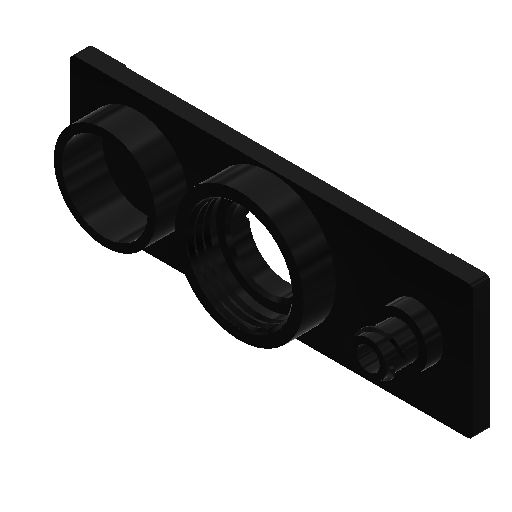
# Autodesk Inventor part: PRT - 9301 - MFLEAFCHIP - V04 - A
Saved by Autodesk Inventor 2025.3 (Build 293356000, 356)
## iProperties
Part Number: PRT - 9301 - MFLEAFCHIP - V04 - A
Material: Generic
Description: Leaf chamber chip A (luer inlet -> chamber -> open reservoir), print in black resin
Document SubType Name: Modeling
Designer: benir
Appearance: Low Gloss - Black
Author: benir
Autodesk Inventor part; units mm, degrees
ref_plane "z = -cs_recess" through (0, 0, -0.25) normal (0, 0, 1) x (1, 0, 0)
sketch "slab sketch" plane through (0, 0, -0.25) normal (0, 0, 1) x (1, 0, 0)
  line L0 (-37.5, -12.5) -> (37.5, -12.5)
  line L1 (37.5, -12.5) -> (37.5, 12.5)
  line L2 (37.5, 12.5) -> (-37.5, 12.5)
  line L3 (-37.5, 12.5) -> (-37.5, -12.5)
  line L4 (0, -17.5) -> (0, 17.5) projected
  line L5 (-52.5, 0) -> (52.5, 0) projected
  dimension "d1" = 75
  dimension "d2" = 25
  constraints: 8 end point, 2 parallel, 1 horizontal, 1 perpendicular, 2 other
  measures "d1" distance of L0.start L0.end
  measures "d2" distance of L2.end L0.start
extrude "slab" add sketch "slab sketch" along normal blind 3.25
fillet "slab corners" radius 1 4 edges at (-37.5, -12.5, 1.375) (-37.5, 12.5, 1.375) (37.5, 12.5, 1.375) (37.5, -12.5, 1.375)
sketch "glue band sketch" plane through (0, 0, 0) normal (0, 0, 1) x (1, 0, 0)
  line L0 (-30.25, -13.5) -> (30.25, -13.5)
  line L1 (30.25, -13.5) -> (30.25, 13.5)
  line L2 (30.25, 13.5) -> (-30.25, 13.5)
  line L3 (-30.25, 13.5) -> (-30.25, -13.5)
  line L4 (0, -18.9) -> (0, 18.9) projected
  line L5 (-52.5, 0) -> (52.5, 0) projected
  dimension "d6" = 60.5
  dimension "d7" = 27
  constraints: 8 end point, 2 parallel, 1 horizontal, 1 perpendicular, 2 other
  measures "d6" distance of L0.start L0.end
  measures "d7" distance of L2.end L0.start
extrude "glue band (bottom coverslip)" cut sketch "glue band sketch" against normal blind 0.75
ref_plane "z = base_t" through (0, 0, 3) normal (0, 0, 1) x (1, 0, 0)
sketch "chamber boss sketch" plane through (0, 0, 3) normal (0, 0, 1) x (1, 0, 0)
  circle A0 centre (0, 0) radius 12
  dimension "d11" = 24
  constraints: 1 centre point
  measures "d11" diameter of A0
extrude "chamber boss" add sketch "chamber boss sketch" along normal blind 6
sketch "reservoir boss sketch" plane through (0, 0, 3) normal (0, 0, 1) x (1, 0, 0)
  circle A0 centre (-25, 0) radius 9.5
  line L0 (-52.5, 0) -> (52.5, 0) projected
  point P0 (0, 0)
  dimension "d14" = 25
  dimension "d15" = 19
  constraints: 1 centre point, 1 point on line
  measures "d14" distance of point (0, 0) A0.centre
  measures "d15" diameter of A0
extrude "reservoir boss" add sketch "reservoir boss sketch" along normal blind 6
sketch "inlet luer foot sketch" plane through (0, 0, 3) normal (0, 0, 1) x (1, 0, 0)
  circle A0 centre (27, 0) radius 5
  line L0 (-52.5, 0) -> (52.5, 0) projected
  point P0 (0, 0)
  dimension "d18" = 27
  dimension "d19" = 10
  constraints: 1 centre point, 1 point on line
  measures "d18" distance of point (0, 0) A0.centre
  measures "d19" diameter of A0
extrude "inlet luer foot" add sketch "inlet luer foot sketch" along normal blind 3
sketch "inlet luer hub sketch" plane through (0, 0, 3) normal (0, 0, 1) x (1, 0, 0)
  circle A0 centre (27, 0) radius 3.365
  line L0 (-52.5, 0) -> (52.5, 0) projected
  point P0 (0, 0)
  dimension "d22" = 27
  dimension "d23" = 6.73
  constraints: 1 centre point, 1 point on line
  measures "d22" distance of point (0, 0) A0.centre
  measures "d23" diameter of A0
extrude "inlet luer hub" add sketch "inlet luer hub sketch" along normal blind 9
ref_plane "x = in_x" through (27, 0, 0) normal (1, 0, 0) x (0, 1, 0)
sketch "inlet luer lug profile" plane through (0, 0, 0) normal (0, 1, 0) x (-1, 0, 0)
  line L0 (-30.265, 8.25) -> (-30.915, 8.55)
  line L1 (-30.915, 8.55) -> (-30.915, 8.9)
  line L2 (-30.915, 8.9) -> (-30.265, 9.2)
  line L3 (-30.265, 9.2) -> (-30.265, 8.25)
  point P0 (0, 0)
  dimension "d27" = 8.25
  dimension "d28" = 30.265
  dimension "d29" = 8.55
  dimension "d30" = 30.915
  dimension "d31" = 8.9
  dimension "d32" = 30.915
  dimension "d33" = 9.2
  dimension "d34" = 30.265
  constraints: 8 end point
  measures "d27" vertical distance of point (0, 0) L0.start
  measures "d28" horizontal distance of point (0, 0) L0.start
  measures "d29" vertical distance of point (0, 0) L0.end
  measures "d30" horizontal distance of point (0, 0) L0.end
  measures "d31" vertical distance of point (0, 0) L1.end
  measures "d32" horizontal distance of point (0, 0) L1.end
  measures "d33" vertical distance of point (0, 0) L2.end
  measures "d34" horizontal distance of point (0, 0) L2.end
coil "inlet luer lug (RH, lead luer_lead)" sketch "inlet luer lug profile" operation add axis through (27, 0, 0) along (0, 0, 1) pitch 5 turns 0.5 hand right
pattern_circular "inlet luer lugs x2" count 2 over 360 about axis through (27, 0, 0) along (0, 0, 1) of "inlet luer lug (RH, lead luer_lead)"
sketch "well sketch" plane through (0, 0, 0) normal (0, 0, 1) x (1, 0, 0)
  circle A0 centre (0, 0) radius 7.15
  dimension "d46" = 14.3
  constraints: 1 centre point
  measures "d46" diameter of A0
extrude "chamber well" cut sketch "well sketch" along normal blind 4
ref_plane "z = ledge_z" through (0, 0, 4) normal (0, 0, 1) x (1, 0, 0)
sketch "thread bore sketch" plane through (0, 0, 4) normal (0, 0, 1) x (1, 0, 0)
  circle A0 centre (0, 0) radius 9.338125
  dimension "d50" = 18.67625
  constraints: 1 centre point
  measures "d50" diameter of A0
extrude "thread bore" cut sketch "thread bore sketch" along normal blind 6
chamfer "thread lead-in" distance 0.6 angle 45 1 edges at (-9.3381, 0, 9)
chamfer "O-ring lead-in" distance 0.6 angle 45 1 edges at (-7.15, 0, 4)
sketch "internal thread groove profile" plane through (0, 0, 0) normal (0, 1, 0) x (-1, 0, 0)
  line L0 (-9.238125, 4.3) -> (-10.15, 4.826471)
  line L1 (-10.15, 4.826471) -> (-10.15, 5.013971)
  line L2 (-10.15, 5.013971) -> (-9.238125, 5.540442)
  line L3 (-9.238125, 5.540442) -> (-9.238125, 4.3)
  point P0 (0, 0)
  dimension "d59" = 4.3
  dimension "d60" = 9.23813
  dimension "d61" = 4.82647
  dimension "d62" = 10.15
  dimension "d63" = 5.01397
  dimension "d64" = 10.15
  dimension "d65" = 5.54044
  dimension "d66" = 9.23813
  constraints: 8 end point
  measures "d59" vertical distance of point (0, 0) L0.start
  measures "d60" horizontal distance of point (0, 0) L0.start
  measures "d61" vertical distance of point (0, 0) L0.end
  measures "d62" horizontal distance of point (0, 0) L0.end
  measures "d63" vertical distance of point (0, 0) L1.end
  measures "d64" horizontal distance of point (0, 0) L1.end
  measures "d65" vertical distance of point (0, 0) L2.end
  measures "d66" horizontal distance of point (0, 0) L2.end
coil "M20x1.5 internal thread (coil cut, RH)" sketch "internal thread groove profile" operation cut axis through (0, 0, -10) along (0, 0, 1) pitch 1.5 turns 3.719853 hand right
ref_plane "z = res_top" through (0, 0, 9) normal (0, 0, 1) x (1, 0, 0)
sketch "reservoir sketch" plane through (0, 0, 9) normal (0, 0, 1) x (1, 0, 0)
  circle A0 centre (-25, 0) radius 8
  line L0 (-52.5, 0) -> (52.5, 0) projected
  point P0 (0, 0)
  dimension "d76" = 25
  dimension "d77" = 16
  constraints: 1 centre point, 1 point on line
  measures "d76" distance of point (0, 0) A0.centre
  measures "d77" diameter of A0
extrude "reservoir" cut sketch "reservoir sketch" against normal blind 7.5
ref_plane "z = luer_top" through (0, 0, 12) normal (0, 0, 1) x (1, 0, 0)
sketch "inlet luer bore sketch" plane through (0, 0, 12) normal (0, 0, 1) x (1, 0, 0)
  circle A0 centre (27, 0) radius 2.145
  line L0 (-52.5, 0) -> (52.5, 0) projected
  point P0 (0, 0)
  dimension "d81" = 27
  dimension "d82" = 4.29
  constraints: 1 centre point, 1 point on line
  measures "d81" distance of point (0, 0) A0.centre
  measures "d82" diameter of A0
sketch "inlet luer bore sketch outline for inlet luer taper bore (6 %)" plane through (0, 0, 12) normal (0, 0, 1) x (1, 0, 0)
  circle A0 centre (27, 0) radius 2.145
extrude "inlet luer taper bore (6 %)" cut sketch "inlet luer bore sketch outline for inlet luer taper bore (6 %)" against normal blind 8 draft -1.71836
ref_plane "z = ch_floor" through (0, 0, 0) normal (0, 0, 1) x (1, 0, 0)
sketch "channel sketch" plane through (0, 0, 0) normal (0, 0, 1) x (1, 0, 0)
  line L0 (3.575, -0.5) -> (27, -0.5)
  line L1 (27, -0.5) -> (27, 0.5)
  line L2 (27, 0.5) -> (3.575, 0.5)
  line L3 (3.575, 0.5) -> (3.575, -0.5)
  line L4 (-52.5, 0) -> (52.5, 0) projected
  line L5 (-25, -0.5) -> (-3.575, -0.5)
  line L6 (-3.575, -0.5) -> (-3.575, 0.5)
  line L7 (-3.575, 0.5) -> (-25, 0.5)
  line L8 (-25, 0.5) -> (-25, -0.5)
  point P0 (0, 0)
  dimension "d86" = 1
  dimension "d87" = 3.575
  dimension "d88" = 27
  dimension "d89" = 1
  dimension "d90" = 25
  dimension "d91" = 3.575
  constraints: 16 end point, 4 parallel, 2 horizontal, 2 perpendicular, 2 other
  measures "d86" distance of L2.end L0.start
  measures "d87" horizontal distance of point (0, 0) L2.end
  measures "d88" horizontal distance of point (0, 0) L0.end
  measures "d89" distance of L7.end L5.start
  measures "d90" horizontal distance of point (0, 0) L7.end
  measures "d91" horizontal distance of point (0, 0) L5.end
extrude "channels" cut sketch "channel sketch" along normal blind 0.5
sketch "inlet via sketch" plane through (0, 0, 0) normal (0, 0, 1) x (1, 0, 0)
  circle A0 centre (27, 0) radius 0.5
  line L0 (-52.5, 0) -> (52.5, 0) projected
  point P0 (0, 0)
  dimension "d94" = 27
  dimension "d95" = 1
  constraints: 1 centre point, 1 point on line
  measures "d94" distance of point (0, 0) A0.centre
  measures "d95" diameter of A0
extrude "inlet via" cut sketch "inlet via sketch" along normal blind 4.3
sketch "outlet via sketch" plane through (0, 0, 0) normal (0, 0, 1) x (1, 0, 0)
  circle A0 centre (-25, 0) radius 0.5
  line L0 (-52.5, 0) -> (52.5, 0) projected
  point P0 (0, 0)
  dimension "d98" = 25
  dimension "d99" = 1
  constraints: 1 centre point, 1 point on line
  measures "d98" distance of point (0, 0) A0.centre
  measures "d99" diameter of A0
extrude "outlet via" cut sketch "outlet via sketch" along normal blind 1.8
equation "\"d1\" = chip_l"
equation "\"d2\" = chip_w"
equation "\"d3\" = base_t + cs_recess"
equation "\"d5\" = corner_r"
equation "\"d6\" = cs_l + 2 * cs_gap"
equation "\"d11\" = boss_d"
equation "\"d12\" = boss_top - base_t"
equation "\"d14\" = out_x"
equation "\"d15\" = res_d + 2 * res_wall"
equation "\"d16\" = res_top - base_t"
equation "\"d18\" = in_x"
equation "\"d19\" = luer_foot_d"
equation "\"d20\" = -luer_free + luer_top - base_t"
equation "\"d22\" = in_x"
equation "\"d23\" = luer_hub_d"
equation "\"d24\" = luer_top - base_t"
equation "\"d27\" = lug_zc - 0.5 * luer_lug_base"
equation "\"d28\" = in_x + lug_r_in"
equation "\"d29\" = lug_zc - 0.5 * luer_lug_crest"
equation "\"d30\" = in_x + 0.5 * luer_lug_d"
equation "\"d31\" = lug_zc + 0.5 * luer_lug_crest"
equation "\"d32\" = in_x + 0.5 * luer_lug_d"
equation "\"d33\" = lug_zc + 0.5 * luer_lug_base"
equation "\"d34\" = in_x + lug_r_in"
equation "\"d35\" = luer_lead"
equation "\"d37\" = luer_lug_rev"
equation "\"d46\" = well_d"
equation "\"d47\" = ledge_z"
equation "\"d50\" = th_bore_d"
equation "\"d53\" = th_chamfer"
equation "\"d54\" = th_chamfer"
equation "\"d56\" = well_chamfer"
equation "\"d57\" = well_chamfer"
equation "\"d59\" = ti_zc - 0.5 * ti_w_in"
equation "\"d60\" = ti_r_in"
equation "\"d61\" = ti_zc - 0.5 * ti_w_root"
equation "\"d62\" = 0.5 * th_root_d"
equation "\"d63\" = ti_zc + 0.5 * ti_w_root"
equation "\"d64\" = 0.5 * th_root_d"
equation "\"d65\" = ti_zc + 0.5 * ti_w_in"
equation "\"d66\" = ti_r_in"
equation "\"d67\" = th_p"
equation "\"d68\" = ti_height"
equation "\"d76\" = out_x"
equation "\"d77\" = res_d"
equation "\"d78\" = res_top - res_floor"
equation "\"d81\" = in_x"
equation "\"d82\" = luer_open_d"
equation "\"d83\" = luer_depth"
equation "\"d84\" = -luer_taper_deg"
equation "\"d86\" = ch_w"
equation "\"d87\" = 0.25 * well_d"
equation "\"d88\" = in_x"
equation "\"d89\" = ch_w"
equation "\"d90\" = out_x"
equation "\"d91\" = 0.25 * well_d"
equation "\"d92\" = ch_h"
equation "\"d94\" = in_x"
equation "\"d95\" = via_d"
equation "\"d98\" = out_x"
equation "\"d99\" = via_d"
equation "\"cs_recess\" = 0.25"
equation "\"d0\" = -cs_recess"
equation "\"chip_l\" = 75"
equation "\"chip_w\" = 25"
equation "\"base_t\" = 3"
equation "\"corner_r\" = 1"
equation "\"cs_gap\" = 0.25"
equation "\"d10\" = base_t"
equation "\"boss_d\" = 24"
equation "\"chamber_h\" = 0.8"
equation "\"stub_len\" = 3.2"
equation "\"ledge_z\" = chamber_h + stub_len"
equation "\"th_len\" = 5"
equation "\"boss_top\" = ledge_z + th_len"
equation "\"out_x\" = 25"
equation "\"res_d\" = 16"
equation "\"res_wall\" = 1.5"
equation "\"res_top\" = 9"
equation "\"in_x\" = 27"
equation "\"luer_foot_d\" = 10"
equation "\"luer_top\" = 12"
equation "\"luer_free\" = 6"
equation "\"luer_hub_d\" = 6.73"
equation "\"d26\" = in_x"
equation "\"luer_lug_gap\" = 0.3"
equation "\"luer_lug_base\" = 0.95"
equation "\"luer_lug_rev\" = 0.5"
equation "\"luer_lead\" = 5"
equation "\"luer_lug_d\" = 7.83"
equation "\"luer_lug_crest\" = 0.35"
equation "\"well_d\" = 14.3"
equation "\"d49\" = ledge_z"
equation "\"th_p\" = 1.5"
equation "\"th_clear\" = 0.15"
equation "\"th_bore_d\" = -1.0825 * th_p + th_d + 2 * th_clear"
equation "\"th_chamfer\" = 0.6"
equation "\"well_chamfer\" = 0.6"
equation "\"th_start\" = 0.3"
equation "\"ti_w_root\" = 0.125 * th_p"
equation "\"th_root_d\" = th_d + 2 * th_clear"
equation "\"ti_w_in\" = ti_w_root + 0.57735 * th_root_d - 1.1547 * ti_r_in"
equation "\"ti_zc\" = th_start + ledge_z + 0.5 * ti_w_in"
equation "\"ti_height\" = th_p + boss_top - ti_zc"
equation "\"d75\" = res_top"
equation "\"res_floor\" = 1.5"
equation "\"d80\" = luer_top"
equation "\"luer_open_d\" = 4.29"
equation "\"luer_depth\" = 8"
equation "\"luer_taper_deg\" = 1.71836deg"
equation "\"ch_floor\" = 0"
equation "\"ch_w\" = 1"
equation "\"ch_h\" = 0.5"
equation "\"via_d\" = 1"
equation "\"luer_bot_z\" = luer_top - luer_depth"
equation "\"cs_l\" = 60"
equation "\"th_d\" = 20"
equation "\"ti_r_in\" = 9.238125"
equation "\"lug_zc\" = 8.725"
equation "\"lug_r_in\" = 3.265"
body "Solid1"
